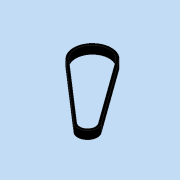
# Autodesk Inventor part: Pas zębaty 10 T5-305
Saved by Autodesk Inventor 2018 (Build 220112000, 112)
## iProperties
Created: 2019-01-31
Part Number: Pas zębaty 10 T5-305
Material: Ogólny
Document SubType Name: Modeling
Designer: Dawid
Density: 1 g/cm^3
Appearance: Anodowana - czarna
Author: Dawid
Autodesk Inventor part; units mm, degrees
ref_plane "YZ Plane" through (0, 0, 0) normal (1, 0, 0) x (0, 1, 0)
ref_plane "XZ Plane" through (0, 0, 0) normal (0, 1, 0) x (-1, 0, 0)
ref_plane "XY Plane" through (0, 0, 0) normal (0, 0, 1) x (1, 0, 0)
sketch "Szkic1" plane through (0, 0, 0) normal (0, 0, 1) x (1, 0, 0)
  line L0 (-44.1102, 22.1496) -> (-6.9652, -10.0467)
  line L1 (-44.1102, 22.1496) -> (-82.1839, 55.1508)
  line L2 (-16.9855, 44.2353) -> (-47.7027, 86.7194)
  line L3 (-16.9855, 44.2353) -> (10.6211, 6.0535)
  arc A0 (-47.7027, 86.7194) -> (-82.1839, 55.1508) centre (-65.0027, 71) ccw
  arc A1 (-6.9652, -10.0467) -> (10.6211, 6.0535) centre (0, 0) ccw
  line L4 (-19.1735, 42.6533) -> (4.6935, 9.6435)
  line L5 (-42.3418, 24.1898) -> (-70.0034, 48.1662)
  line L6 (-42.3418, 24.1898) -> (-10.0192, -3.8265)
  line L7 (-19.1735, 42.6533) -> (-41.8174, 73.9714)
  arc A2 (-48.3661, 83.0288) -> (-78.4492, 55.4867) centre (-65.0027, 71) ccw
  line L8 (-41.8174, 73.9714) -> (-48.3661, 83.0288)
  line L9 (-70.0034, 48.1662) -> (-78.4492, 55.4867)
  arc A3 (-6.4825, -6.8812) -> (7.6611, 5.5392) centre (0, 0) ccw
  line L10 (4.6935, 9.6435) -> (7.6611, 5.5392)
  line L11 (-10.0192, -3.8265) -> (-5.865, -7.4145)
  point P0 (0, 0)
  constraints: 27 end point, 9 point on circle, 4 centre point, 1 coincident, 1 point on line
extrude "Wyciągnięcie proste1" add sketch "Szkic1" along normal blind 10
